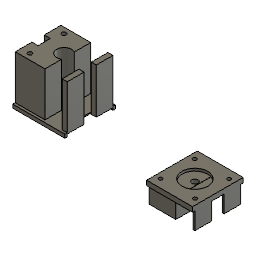
sp-r lite pedal loadcell mount v1 (Autodesk Fusion 360 design; units mm, degrees)
Autodesk Fusion 360 part; units mm, degrees
sketch "スケッチ1" plane through (0, 0, 0) normal (0, 1, 0) x (1, 0, 0)
  line L0 (0, 0) -> (42.5, 0)
  line L1 (42.5, 0) -> (42.5, -37.4)
  line L2 (42.5, -37.4) -> (0, -37.4)
  line L3 (0, -37.4) -> (0, 0)
  line L4 (0, -13.7) -> (0, -23.7)
  line L5 (42.5, -23.7) -> (42.5, -13.7)
  line L6 (16.25, 0) -> (26.25, 0)
  line L7 (26.25, -37.4) -> (16.25, -37.4)
  line L8 (0, 2) -> (42.5, 2)
  line L9 (42.5, 2) -> (42.5, -39.4)
  line L10 (42.5, -39.4) -> (0, -39.4)
  line L11 (0, -39.4) -> (0, 2)
  circle A0 centre (7.2, -4.8) radius 1.75
  circle A1 centre (7.2, -32.6) radius 1.75
  circle A2 centre (21.25, -18.7) radius 6
  line L12 (24.3367, -43.3357) -> (24.3367, 8.7643)
  line L13 (24.3367, 8.7643) -> (38.3367, 8.7643)
  line L14 (38.3367, 8.7643) -> (38.3367, -43.3357)
  line L15 (38.3367, -43.3357) -> (24.3367, -43.3357)
  line L16 (42.5, -23.7) -> (37.5, -23.7)
  line L17 (37.5, -23.7) -> (37.5, -13.7)
  line L18 (37.5, -13.7) -> (42.5, -13.7)
  line L19 (42.5, -13.7) -> (42.5, -23.7)
  line L20 (0, -13.7) -> (5, -13.7)
  line L21 (5, -13.7) -> (5, -23.7)
  line L22 (5, -23.7) -> (0, -23.7)
  line L23 (0, -23.7) -> (0, -13.7)
  circle A3 centre (21.25, -18.7) radius 2.5
  line L24 (5, -13.7) -> (5, -23.7)
  line L25 (0, -37.4) -> (0, 0)
  line L26 (42.5, -39.4) -> (0, -39.4)
  line L27 (37.5, -13.7) -> (42.5, -13.7)
  line L28 (42.5, 0) -> (42.5, -37.4)
  line L29 (16.25, 0) -> (26.25, 0)
  line L30 (37.5, -23.7) -> (37.5, -13.7)
  line L31 (0, 2) -> (42.5, 2)
  line L32 (0, -13.7) -> (0, -23.7)
  line L33 (24.3367, 8.7643) -> (36.4367, 8.7643)
  line L34 (42.5, -13.7) -> (42.5, -23.7)
  line L35 (0, -13.7) -> (5, -13.7)
  line L36 (36.4367, -43.3357) -> (24.3367, -43.3357)
  line L37 (5, -23.7) -> (0, -23.7)
  line L38 (42.5, -23.7) -> (42.5, -13.7)
  circle A4 centre (21.25, -18.7) radius 6
  line L39 (42.5, -37.4) -> (0, -37.4)
  circle A5 centre (21.25, -18.7) radius 2.5
  line L40 (42.5, 2) -> (42.5, -39.4)
  line L41 (24.3367, -43.3357) -> (24.3367, 8.7643)
  line L42 (0, 0) -> (42.5, 0)
  line L43 (0, -39.4) -> (0, 2)
  line L44 (0, -23.7) -> (0, -13.7)
  line L45 (26.25, -37.4) -> (16.25, -37.4)
  line L46 (42.5, -23.7) -> (37.5, -23.7)
  line L47 (108.828, -39.5665) -> (108.828, -2.1665)
  line L48 (108.828, -25.8665) -> (108.828, -15.8665)
  line L49 (108.828, -39.5665) -> (108.828, -2.1665)
  line L50 (151.328, -15.8665) -> (151.328, -25.8665)
  line L51 (151.328, -0.1665) -> (151.328, -41.5665)
  line L52 (108.828, -41.5665) -> (108.828, -0.1665)
  line L53 (108.828, -41.5665) -> (108.828, -0.1665)
  line L54 (147.1647, 6.5977) -> (147.1647, -45.5023)
  circle A6 centre (130.078, -20.8665) radius 6
  line L55 (151.328, -15.8665) -> (151.328, -25.8665)
  circle A7 centre (144.128, -6.9665) radius 1.5
  line L56 (151.328, -25.8665) -> (146.328, -25.8665)
  line L57 (151.328, -25.8665) -> (146.328, -25.8665)
  line L58 (108.828, -2.1665) -> (151.328, -2.1665)
  circle A8 centre (144.128, -34.7665) radius 1.5
  line L59 (151.328, -41.5665) -> (108.828, -41.5665)
  line L60 (151.328, -41.5665) -> (108.828, -41.5665)
  line L61 (108.828, -0.1665) -> (151.328, -0.1665)
  line L62 (151.328, -39.5665) -> (108.828, -39.5665)
  line L63 (135.078, -39.5665) -> (125.078, -39.5665)
  line L64 (135.078, -39.5665) -> (125.078, -39.5665)
  circle A9 centre (130.078, -20.8665) radius 2.5
  circle A10 centre (130.078, -20.8665) radius 2.5
  line L65 (113.828, -25.8665) -> (108.828, -25.8665)
  line L66 (146.328, -15.8665) -> (151.328, -15.8665)
  circle A11 centre (116.028, -6.9665) radius 1.5
  line L67 (108.828, -15.8665) -> (113.828, -15.8665)
  line L68 (125.078, -2.1665) -> (135.078, -2.1665)
  line L69 (133.1647, 6.5977) -> (147.1647, 6.5977)
  line L70 (108.828, -15.8665) -> (113.828, -15.8665)
  line L71 (125.078, -2.1665) -> (135.078, -2.1665)
  line L72 (108.828, -0.1665) -> (151.328, -0.1665)
  line L73 (113.828, -25.8665) -> (108.828, -25.8665)
  line L74 (151.328, -39.5665) -> (108.828, -39.5665)
  circle A12 centre (116.028, -34.7665) radius 1.5
  line L75 (146.328, -15.8665) -> (151.328, -15.8665)
  line L76 (108.828, -15.8665) -> (108.828, -25.8665)
  line L77 (146.328, -25.8665) -> (146.328, -15.8665)
  line L78 (151.328, -2.1665) -> (151.328, -39.5665)
  line L79 (108.828, -25.8665) -> (108.828, -15.8665)
  line L80 (113.828, -15.8665) -> (113.828, -25.8665)
  line L81 (133.1647, -45.5023) -> (133.1647, 6.5977)
  line L82 (146.328, -25.8665) -> (146.328, -15.8665)
  circle A13 centre (130.078, -20.8665) radius 6
  line L83 (151.328, -2.1665) -> (151.328, -39.5665)
  line L84 (151.328, -25.8665) -> (151.328, -15.8665)
  line L85 (108.828, -15.8665) -> (108.828, -25.8665)
  line L86 (151.328, -0.1665) -> (151.328, -41.5665)
  line L87 (113.828, -15.8665) -> (113.828, -25.8665)
  line L88 (151.328, -25.8665) -> (151.328, -15.8665)
  line L89 (133.2647, -45.5023) -> (133.2647, 6.5977)
  line L90 (147.1647, -45.5023) -> (133.1647, -45.5023)
  line L91 (147.2647, 6.5977) -> (147.2647, -45.5023)
  line L92 (147.2647, -45.5023) -> (133.2647, -45.5023)
  line L93 (133.2647, 6.5977) -> (147.2647, 6.5977)
  line L94 (108.828, -2.1665) -> (151.328, -2.1665)
  circle A14 centre (130.078, -20.8665) radius 10.5
  circle A15 centre (31.3367, -18.5855) radius 2
  circle A16 centre (140.1647, -20.7525) radius 2
  line L95 (148.828, -0.1665) -> (148.828, -41.5665)
  line L96 (111.328, -0.1665) -> (111.328, -41.5665)
  point P0 (108.828, -2.1665)
  dimension "d1" = 42.5
  dimension "d2" = 37.4
  dimension "d11" = 41.4
  dimension "d12" = 2
  dimension "d13" = 3.5
  dimension "d14" = 4.8
  dimension "d15" = 7.2
  dimension "d18" = 3.5
  dimension "d20" = 4.8
  dimension "d23" = 21.25
  dimension "d24" = 18.7
  dimension "d25" = 52.1
  dimension "d26" = 14
  dimension "d27" = 5
  dimension "d28" = 10
  dimension "d29" = 5
  dimension "d30" = 10
  dimension "d31" = 5
  dimension "d32" = 12
  dimension "d43" = 42.5
  dimension "d44" = 37.4
  dimension "d45" = 41.4
  dimension "d46" = 2
  dimension "d57" = 21.25
  dimension "d58" = 18.7
  dimension "d59" = 52.1
  dimension "d61" = 5
  dimension "d62" = 10
  dimension "d63" = 5
  dimension "d64" = 10
  dimension "d65" = 5
  dimension "d66" = 12
  dimension "d68" = 37.4
  dimension "d70" = 2
  dimension "d74" = 3
  dimension "d75" = 7.2
  dimension "d76" = 3
  dimension "d77" = 3
  dimension "d78" = 4.8
  dimension "d79" = 4.8
  dimension "d80" = 4.8
  dimension "d81" = 21.25
  dimension "d83" = 52.1
  dimension "d91" = 42.5
  dimension "d93" = 41.4
  dimension "d95" = 3
  dimension "d96" = 4.8
  dimension "d97" = 7.2
  dimension "d106" = 18.7
  dimension "d109" = 5
  dimension "d110" = 10
  dimension "d111" = 5
  dimension "d112" = 10
  dimension "d113" = 5
  dimension "d114" = 12
  dimension "d115" = 21
  dimension "d130" = 4
  dimension "d131" = 7
  dimension "d132" = 4
  dimension "d133" = 7
  dimension "d134" = 20.8145
  dimension "d136" = 20.814
  dimension "d139" = 4.1633
  dimension "d140" = 4.1633
  dimension "d141" = 2.5
  dimension "d142" = 2.5
  constraint horizontal L0
  constraint vertical L1
  constraint horizontal L2
  constraint vertical L3
  constraint coincident L0.start L3.end
  constraint vertical L4
  constraint vertical L5
  constraint coincident L3 L4.end
  constraint coincident L1 L5.end
  constraint horizontal L6
  constraint horizontal L7
  constraint coincident L2 L7.start
  constraint coincident L0 L6.start
  constraint horizontal L8
  constraint vertical L9
  constraint horizontal L10
  constraint vertical L11
  constraint coincident L1 L9.end
  constraint horizontal L16
  constraint vertical L17
  constraint horizontal L18
  constraint vertical L19
  constraint midpoint L9 L19
  constraint horizontal L20
  constraint vertical L21
  constraint horizontal L22
  constraint vertical L23
  constraint midpoint L11 L23
  constraint concentric A2 A3
  constraint horizontal L42
  constraint vertical L28
  constraint horizontal L39
  constraint vertical L25
  constraint vertical L32
  constraint vertical L38
  constraint coincident L4.end L25
  constraint coincident L5.end L28
  constraint horizontal L29
  constraint horizontal L45
  constraint coincident L7.start L39
  constraint coincident L6.start L42
  constraint horizontal L31
  constraint vertical L40
  constraint horizontal L26
  constraint vertical L43
  constraint coincident L9.end L28
  constraint horizontal L46
  constraint vertical L30
  constraint horizontal L27
  constraint vertical L34
  constraint midpoint L34 L40
  constraint horizontal L35
  constraint vertical L24
  constraint horizontal L37
  constraint vertical L44
  constraint midpoint L43 L44
  constraint concentric A4 A5
  constraint horizontal L58
  constraint vertical L78
  constraint horizontal L62
  constraint vertical L49
  constraint vertical L85
  constraint vertical L88
  constraint coincident L48.start L49
  constraint coincident L50.start L78
  constraint horizontal L71
  constraint horizontal L64
  constraint coincident L63.start L62
  constraint coincident L68.start L58
  constraint horizontal L72
  constraint vertical L86
  constraint horizontal L59
  constraint vertical L52
  constraint coincident L51.end L78
  constraint horizontal L56
  constraint vertical L82
  constraint horizontal L66
  constraint vertical L50
  constraint midpoint L50 L86
  constraint horizontal L70
  constraint vertical L80
  constraint horizontal L73
  constraint vertical L48
  constraint midpoint L48 L52
  constraint concentric A10 A13
  constraint horizontal L94
  constraint vertical L83
  constraint horizontal L74
  constraint vertical L47
  constraint coincident P0 L47.end
  constraint vertical L76
  constraint vertical L84
  constraint coincident L48.start L47
  constraint coincident L50.start L83
  constraint horizontal L68
  constraint horizontal L63
  constraint coincident L63.start L74
  constraint coincident L68.start L94
  constraint horizontal L61
  constraint vertical L51
  constraint horizontal L60
  constraint vertical L53
  constraint coincident L51.end L83
  constraint horizontal L57
  constraint vertical L77
  constraint horizontal L75
  constraint vertical L55
  constraint midpoint L51 L55
  constraint horizontal L67
  constraint vertical L87
  constraint horizontal L65
  constraint vertical L79
  constraint midpoint L53 L79
  constraint concentric A6 A9
  constraint concentric A6 A14
  constraint coincident L61 L95.start
  constraint coincident L59 L95.end
  constraint perpendicular L59 L95
  constraint coincident L61 L96.start
  constraint coincident L59 L96.end
  constraint perpendicular L59 L96
  measures "d1" distance of L0.start L0.end
  measures "d2" distance of L0.start L2.end
  measures "d11" distance of L8 L10
  measures "d12" distance of L0 L8
  measures "d13" diameter of A0
  measures "d14" distance of L0 A0.centre
  measures "d15" distance of L3 A0.centre
  measures "d18" diameter of A1
  measures "d20" distance of L2 A1.centre
  measures "d23" distance of L11 A2.centre
  measures "d24" distance of L6 A2.centre
  measures "d25" distance of L12.start L12.end
  measures "d26" distance of L12.start L14.end
  measures "d27" distance of L5.start L16.end
  measures "d28" distance of L5.start L5.end
  measures "d29" distance of L4.start L20.end
  measures "d30" distance of L4.start L4.end
  measures "d31" diameter of A3
  measures "d32" diameter of A2
  measures "d43" distance of L0.start L0.end
  measures "d44" distance of L2.end L0.start
  measures "d45" distance of L26 L31
  measures "d46" distance of L31 L42
  measures "d57" distance of A2.centre L43
  measures "d58" distance of A2.centre L29
  measures "d59" distance of L12.start L12.end
  measures "d61" distance of L16.end L5.start
  measures "d62" distance of L5.start L5.end
  measures "d63" distance of L20.end L4.start
  measures "d64" distance of L4.end L4.start
  measures "d65" diameter of A5
  measures "d66" diameter of A4
  measures "d68" distance of L47.start P0
  measures "d70" distance of L58 L72
  measures "d74" diameter of A7
  measures "d75" distance of A7.centre L78
  measures "d76" diameter of A12
  measures "d77" diameter of A8
  measures "d78" distance of A12.centre L62
  measures "d79" distance of A8.centre L62
  measures "d80" distance of A7.centre L58
  measures "d81" distance of A6.centre L52
  measures "d83" distance of L81.start L69.start
  measures "d91" distance of L58.end P0
  measures "d93" distance of L60 L61
  measures "d95" diameter of A11
  measures "d96" distance of A11.centre L94
  measures "d97" distance of A11.centre L47
  measures "d106" distance of A6.centre L68
  measures "d109" distance of L56.end L50.end
  measures "d110" distance of L50.start L50.end
  measures "d111" distance of L48.end L67.end
  measures "d112" distance of L48.end L48.start
  measures "d113" diameter of A9
  measures "d114" diameter of A6
  measures "d115" diameter of A14
  measures "d130" diameter of A15
  measures "d131" distance of L12 A15.centre
  measures "d132" diameter of A16
  measures "d133" distance of L81 A16.centre
  measures "d134" distance of L10 A15.centre
  measures "d136" distance of L59 A16.centre
  measures "d139" distance of L9 L14
  measures "d140" distance of L51 L54
  measures "d141" distance of L51 L95
  measures "d142" distance of L52 L96
extrude "押し出し1" add sketch "スケッチ1" along normal blind 1 contours L0 L2 L3 L6 L7 L11 A2 L12 L20 L21 L22 L24 L25 L29 L35 L37 A4 L39 L41 L42 L43 L45 | L0 L2 L6 L7 A2 L12 L14 L16 L17 L18 L27 L29 L30 A4 L39 L41 L42 L45 L46 | L0 L1 L9 L14 L18 L27 L28 L40 L42 | L1 L2 L9 L14 L16 L28 L39 L40 L46 | A15 makes body 1
extrude "押し出し2" add sketch "スケッチ1" along normal blind 1 and the other way blind 2 contours L0 L6 L8 L11 L12 L29 L31 L41 L42 L43 | L0 L6 L8 L12 L14 L29 L31 L41 L42 | A2 L12 A4 L41 | A2 L12 A4 L41 | L2 L7 L10 L11 L12 L26 L39 L41 L43 L45 | L0 L8 L9 L14 L31 L40 L42 | L2 L7 L10 L12 L14 L26 L39 L41 L45 | L2 L9 L10 L14 L26 L39 L40 bodies 1
extrude "押し出し3" add sketch "スケッチ1" along normal blind 1 separate body contours L0 L2 L3 L6 L7 L11 A2 L12 L20 L21 L22 L24 L25 L29 L35 L37 A4 L39 L41 L42 L43 L45 | L0 L2 L6 L7 A2 L12 L14 L16 L17 L18 L27 L29 L30 A4 L39 L41 L42 L45 L46 | A2 L12 A4 L41 | A2 L12 A4 L41 | L0 L1 L9 L14 L18 L27 L28 L40 L42 | L1 L2 L9 L14 L16 L28 L39 L40 L46 | A15 makes body 2
extrude "押し出し4" add sketch "スケッチ1" along normal blind 37 contours L0 L2 L3 L6 L7 L11 A2 L12 L20 L21 L22 L24 L25 L29 L35 L37 A4 L39 L41 L42 L43 L45 | L0 L1 L9 L14 L18 L27 L28 L40 L42 | L1 L2 L9 L14 L16 L28 L39 L40 L46 bodies 2 1
extrude "押し出し5" add sketch "スケッチ1" along normal blind 2 separate body contours L59 L60 L62 L63 L64 L74 L81 L96 | L58 L61 L68 L71 L72 L81 L94 L96 | L59 L60 L62 L74 L91 L95 | L58 L61 L72 L91 L94 L95 makes body 3 at (148.828, 0.6667, 0.8332) makes body 4 at (147.2647, 0.6667, 40.2332) makes body 5 at (118.6069, 0.6667, 0.1665) makes body 6 at (125.8858, 0.6667, 39.5665)
extrude "押し出し6" add sketch "スケッチ1" along normal blind 2 contours L58 L62 L63 L64 L65 L67 L68 L70 L71 L73 L74 L80 L81 L87 L94 A14 L96 | L59 L60 L62 L63 L64 L74 L81 L96 | L58 L61 L68 L71 L72 L81 L94 L96 | A6 L81 A13 A14 | A6 L81 A13 | L59 L60 L62 L74 L91 L95 | L58 L61 L72 L91 L94 L95 | L58 L66 L75 L91 L94 L95 bodies 3 5 4 6
extrude "押し出し7" add sketch "スケッチ1" along normal blind 2 contours L65 L67 L70 L73 L80 L87 L96 | L54 L56 L57 L66 L75 L77 L82 | L54 L56 L57 L66 L75 L91 | L56 L57 L66 L75 L91 L95 bodies 3 5
extrude "押し出し8" add sketch "スケッチ1" along normal blind 2 contours L54 L59 L60 L62 L63 L64 L74 L89 | L54 L56 L57 L58 L62 L63 L64 L66 L68 L71 L74 L75 L77 L82 L89 L94 A14 A16 | A6 A13 L89 A14 A16 | A6 A13 L89 | A14 A16 | A14 A16 | L54 L58 L61 L68 L71 L72 L89 L94 | L54 L56 L57 L66 L75 L77 L82 bodies 3 4 5
extrude "押し出し9" add sketch "スケッチ1" along normal blind 4 contours L58 L62 L63 L64 L65 L67 L68 L70 L71 L73 L74 L80 L81 L87 L94 A14 L96 | L59 L60 L62 L63 L64 L74 L81 L96 | L65 L67 L70 L73 L80 L87 L96 | L59 L60 L62 L63 L64 L74 L81 L89 | L62 L63 L64 L74 L81 L89 A14 | L58 L61 L68 L71 L72 L81 L94 L96 | L54 L59 L60 L62 L63 L64 L74 L89 | L54 L56 L57 L58 L62 L63 L64 L66 L68 L71 L74 L75 L77 L82 L89 L94 A14 A16 | L54 L59 L60 L62 L74 L91 | L58 L68 L71 L81 L89 L94 A14 | L58 L61 L68 L71 L72 L81 L89 L94 | L54 L56 L57 L62 L74 L91 | L59 L60 L62 L74 L91 L95 | A14 A16 | L54 L58 L61 L68 L71 L72 L89 L94 | L54 L56 L57 L66 L75 L77 L82 | L54 L56 L57 L66 L75 L91 | L56 L57 L62 L74 L91 L95 | L54 L58 L61 L72 L91 L94 | L54 L58 L66 L75 L91 L94 | L56 L57 L66 L75 L91 L95 | L58 L61 L72 L91 L94 L95 | L58 L66 L75 L91 L94 L95 picked at (141.0704, -20.4001) bodies 3 5 4
extrude "押し出し10" add sketch "スケッチ1" against normal blind 14 contours L58 L62 L63 L64 L65 L67 L68 L70 L71 L73 L74 L80 L81 L87 L94 A14 L96 | A6 L81 A13 A14 | A6 L81 A13 | L56 L57 L62 L74 L91 L95 | L58 L66 L75 L91 L94 L95 bodies 3
extrude "押し出し11" add sketch "スケッチ1" against normal blind 8 contours A14 A16 | A14 A16 bodies 3
extrude "押し出し12" add sketch "スケッチ1" along normal blind 8 contours A15 bodies 2
equation "d23 = ( 42.5 / 2 ) * 1 mm"
equation "d24 = ( 37.4 / 2 ) * 1 mm"
equation "d57 = ( 42.5 / 2 ) * 1 mm"
equation "d58 = ( 37.4 / 2 ) * 1 mm"
equation "d81 = ( 42.5 / 2 ) * 1 mm"
equation "d106 = ( 37.4 / 2 ) * 1 mm"
named bodies: "bottom", "top"
